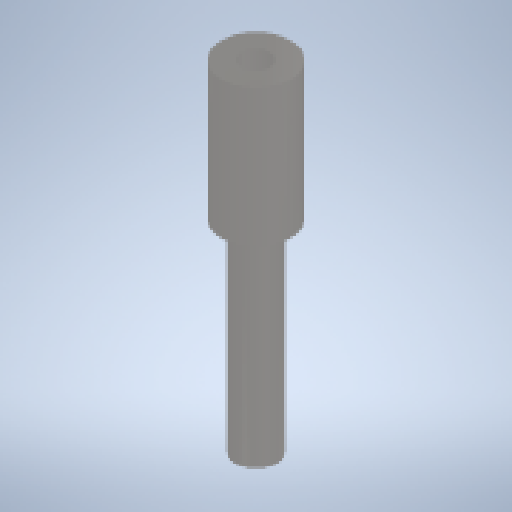
# Autodesk Inventor part: 041
Saved by Autodesk Inventor 2023 (Build 270158000, 158)
## iProperties
Created: 2022-05-02
Part Number: 041
Material: Stainless Steel, Austenitic
Document SubType Name: Modeling
Designer: vmiguel
Density: 8 g/cm^3
Appearance: Semi-Polished
Author: vmiguel
Autodesk Inventor part; units mm, degrees
ref_plane "YZ Plane" through (0, 0, 0) normal (1, 0, 0) x (0, 1, 0)
ref_plane "XZ Plane" through (0, 0, 0) normal (0, 1, 0) x (-1, 0, 0)
ref_plane "XY Plane" through (0, 0, 0) normal (0, 0, 1) x (1, 0, 0)
sketch "Sketch1" plane through (0, 0, 0) normal (1, 0, 0) x (0, 1, 0)
  line L0 (0, 0) -> (-48, 0)
  line L1 (-10, 0) -> (-10, -1)
  line L2 (-10, -1) -> (0, -1)
  line L3 (0, -1) -> (0, -2.5)
  line L4 (0, -2.5) -> (-14, -2.5)
  line L5 (-14, -2.5) -> (-14, -1.5)
  line L6 (-14, -1.5) -> (-48, -1.5)
  line L7 (-48, -1.5) -> (-48, 0)
  point P0 (-10, -0.5)
  point P1 (-14, -2)
  dimension "d0" = 3
  dimension "d1" = 2
  dimension "d2" = 5
  dimension "d3" = 14
  dimension "d4" = 10
  dimension "d6" = 34
  constraints: 16 end point, 6 perpendicular, 2 midpoint, 1 horizontal, 1 point on line, 1 vertical, 1 vertical alignment
  measures "d0" diameter of L6 L0
  measures "d1" diameter of L2 L0
  measures "d2" diameter of L4 L0
  measures "d3" distance of L3.end L4.end
  measures "d4" horizontal distance of L0.start point (-10, -0.5)
  measures "d6" horizontal distance of L6.end point (-14, -2)
revolve "Revolution1" add sketch "Sketch1" angle 360 about axis through (0, 0, 0) along (0, -1, 0)
thread "Thread1" size "M3x0.5" class "6g" standard "ANSI Metric M Profile" length 5
body "Solid1"
